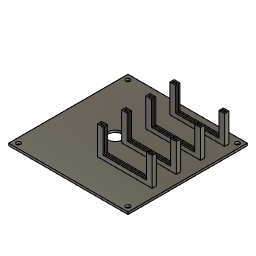
electronics-rack (Autodesk Fusion 360 design; units mm, degrees)
Autodesk Fusion 360 part; units mm, degrees
note: some values were not read from the file. Chosen so that the rebuilt part matches the saved one: which face or edge a step refers to.
box "BoxPrimitive1" add length 84 width 84 height 1.5 placed x (0, 1, 0) y (-1, 0, 0) z (0, 0, 1) at (29, -35, 0) makes body 1
move_body "Move1" bodies 1 to x (1, 0, 0) y (0, 1, 0) z (0, 0, 1) at (-29, 35, 0)
move_body "Move2" bodies 1 to x (1, 0, 0) y (0, 1, 0) z (0, 0, 1) at (42, -42, 0)
box "BoxPrimitive3" add length 3 width 4 height 20 placed x (0, -1, 0) y (1, 0, 0) z (0, 0, 1) at (36, 75, 0) separate body makes body 2
copy_body "CopyPasteBodies1" bodies 2 makes body 3
move_body "Move3" bodies 3 to x (1, 0, 0) y (0, 1, 0) z (0, 0, 1) at (-36.5, 0, 0)
box "BoxPrimitive4" add length 3 width 32.5 height 3 placed x (0, 1, 0) y (-1, 0, 0) z (0, 0, 1) at (36, 72, 0) bodies 2 3
box "BoxPrimitive5" cut length 1 width 36.5 height -25 placed x (0, -1, 0) y (1, 0, 0) z (0, 0, 1) at (2.5, 74, 20) bodies 2
move_face "OffsetFaces1" offset 2 1 faces at (3.5, 72.3333, 8.6667) on bodies 2
move_face "OffsetFaces2" offset 2 1 faces at (3.5, 74.6667, 14.3333) on bodies 2
move_face "OffsetFaces3" offset -2 1 faces at (-0.5, 73, 6.6667) on bodies 2
move_body "Move4" bodies 2 to x (1, 0, 0) y (0, 1, 0) z (0, 0, 1) at (1.5, -38, 0)
move_body "Move5" bodies 2 to x (1, 0, 0) y (0, 1, 0) z (0, 0, 1) at (0, 0, 20)
move_body "Move6" bodies 2 to x (1, 0, 0) y (0, 1, 0) z (0, 0, 1) at (0, 0, 1.5)
move_body "Move7" bodies 2 to x (1, 0, 0) y (0, 1, 0) z (0, 0, 1) at (-1, 3.5, 0)
move_body "Move8" bodies 2 to x (1, 0, 0) y (0, 1, 0) z (0, 0, 1) at (-5, -5, 0)
move_body "Move9" bodies 2 to x (1, 0, 0) y (0, 1, 0) z (0, 0, 1) at (0, 0, -20)
cylinder "CylinderPrimitive1" add diameter 3 height 2 placed x (1, 0, 0) y (0, 1, 0) z (0, 0, 1) at (-42, 42, 0) separate body makes body 4
move_body "Move10" bodies 4 to x (1, 0, 0) y (0, 1, 0) z (0, 0, 1) at (1.5, -1.5, 0)
move_body "Move11" bodies 4 to x (1, 0, 0) y (0, 1, 0) z (0, 0, 1) at (2, -2, 0)
mirror "Mirror1" about plane through (0, 0, 0) normal (1, 0, 0) of bodies 4 makes body 5
mirror "Mirror2" about plane through (0, 0, 0) normal (0, 1, 0) of bodies 4 5 makes body 6 at (-39.8822, -37.9173, 0.6667) makes body 7 at (39.8822, -37.9173, 0.6667)
combine "Combine1" operation cut target body 1 tool bodies 4 7 5 6
move_body "Move12" bodies 2 to x (1, 0, 0) y (0, 1, 0) z (0, 0, 1) at (0.5, -0.5, 0)
copy_body "CopyPasteBodies2" bodies 2 makes body 8
move_body "Move13" bodies 8 to x (1, 0, 0) y (0, 1, 0) z (0, 0, 1) at (0, -17, 0)
copy_body "CopyPasteBodies3" bodies 8 makes body 9
move_body "Move14" bodies 9 to x (1, 0, 0) y (0, 1, 0) z (0, 0, 1) at (0, -17, 0)
copy_body "CopyPasteBodies4" bodies 9 makes body 10
move_body "Move15" bodies 10 to x (1, 0, 0) y (0, 1, 0) z (0, 0, 1) at (0, -17, 0)
cylinder "CylinderPrimitive2" add diameter 10 height 2 placed x (1, 0, 0) y (0, 1, 0) z (0, 0, 1) at (0, 0, 1.5) separate body makes body 11
move_body "Move16" bodies 11 to x (1, 0, 0) y (0, 1, 0) z (0, 0, 1) at (-9, 0, 0)
move_face "OffsetFaces4" offset 9 1 faces at (-7.6899, -1.9935, 3.5) on bodies 11
move_body "Move17" bodies 11 to x (1, 0, 0) y (0, 1, 0) z (0, 0, 1) at (0, 0, -6)
combine "Combine2" operation cut target body 1 tool bodies 11
combine "Combine3" operation add target body 1 tool bodies 2 8 9 10
named bodies: "controller-rack"
